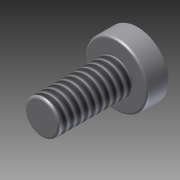
# Autodesk Inventor part: 20mm T-Nut Fastener 1764
Saved by Autodesk Inventor 2011 (Build 150239000, 239)
## iProperties
Created: 2011-02-16
Part Number: 20mm T-Nut Fastener 1764
Document SubType Name: Modeling
Designer: dfranz
Density: 1 g/cm^3
Author: dfranz
Autodesk Inventor part; units mm, degrees
ref_plane "YZ Plane" through (0, 0, 0) normal (1, 0, 0) x (0, 1, 0)
ref_plane "XZ Plane" through (0, 0, 0) normal (0, 1, 0) x (-1, 0, 0)
ref_plane "XY Plane" through (0, 0, 0) normal (0, 0, 1) x (1, 0, 0)
sketch "Sketch1" plane through (0, 0, 0) normal (0, 0, 1) x (1, 0, 0)
  circle A0 centre (0, 0) radius 3.4925
  dimension "d0" = 6.985
  constraints: 1 centre point, 1 coincident
  measures "d0" diameter of A0
extrude "Extrusion1" add sketch "Sketch1" along normal blind 2.54
sketch "Sketch2" plane through (0, 0, 2.54) normal (0, 0, 1) x (1, 0, 0)
  circle A0 centre (0, 0) radius 3.4925 projected
  circle A1 centre (0, 0) radius 1.905
  dimension "d3" = 3.81
  constraints: 1 centre point, 1 coincident
  measures "d3" diameter of A1
extrude "Extrusion2" add sketch "Sketch2" along normal blind 8.255 contours A1
sketch "Sketch3" plane through (0, 0, 0) normal (0, 0, -1) x (-1, 0, 0)
  circle A0 centre (0, 0) radius 3.4925 projected
  line L0 (1.4665, 0) -> (0.7332, -1.27)
  line L1 (0.7332, -1.27) -> (-0.7332, -1.27)
  line L2 (-0.7332, -1.27) -> (-1.4665, 0)
  line L3 (-1.4665, 0) -> (-0.7332, 1.27)
  line L4 (-0.7332, 1.27) -> (0.7332, 1.27)
  line L5 (0.7332, 1.27) -> (1.4665, 0)
  dimension "d6" = 2.54
  constraints: 12 end point, 1 coincident, 13 other
  measures "d6" distance between parallel lines of L1 L4
extrude "Extrusion3" cut sketch "Sketch3" against normal blind 2.54 contours L0 L1 L2 L3 L4 L5
thread "Thread1" size "8-32 UNC" class "2A" standard "ANSI Unified Screw Threads" full length
fillet "Fillet1" radius 0.254 3 edges at (-3.4925, 0, 0) (-3.4925, 0, 2.54) (-1.905, 0, 10.795)
body "Solid1"
